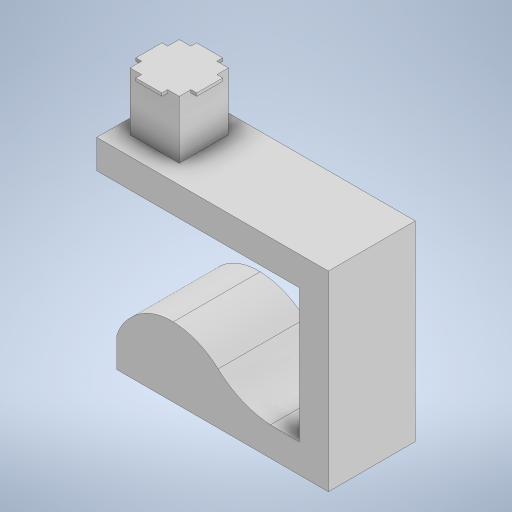
# Autodesk Inventor part: GroundClipV1
Saved by Autodesk Inventor 2024.2 (Build 282272000, 272)
## iProperties
Created: 2024-01-05
Part Number: GroundClipV1
Material: Generic
Document SubType Name: Modeling
Designer: chris
Density: 1 g/cm^3
Appearance: Default
Author: chris
Autodesk Inventor part; units mm, degrees
ref_plane "YZ Plane" through (0, 0, 0) normal (1, 0, 0) x (0, 1, 0)
ref_plane "XZ Plane" through (0, 0, 0) normal (0, 1, 0) x (-1, 0, 0)
ref_plane "XY Plane" through (0, 0, 0) normal (0, 0, 1) x (1, 0, 0)
sketch "Sketch1" plane through (0, 0, 0) normal (0, 1, 0) x (-1, 0, 0)
  line L0 (-20, -7.5) -> (20, -7.5)
  line L1 (20, -7.5) -> (20, 7.5)
  line L2 (20, 7.5) -> (-20, 7.5)
  line L3 (-20, 7.5) -> (-20, -7.5)
  line L4 (-20, -7.5) -> (20, 7.5) construction
  line L5 (20, -7.5) -> (-20, 7.5) construction
  point P0 (0, 0)
  dimension "d0" = 15
  dimension "d1" = 40
  constraints: 12 end point, 2 midpoint, 2 parallel, 1 horizontal, 1 perpendicular
  measures "d0" distance of L0.end L1.end
  measures "d1" distance between parallel lines of L3 L1
extrude "Extrusion1" add sketch "Sketch1" along normal blind 5
sketch "Sketch2" plane through (20, 0, 7.5) normal (1, 0, 0) x (0, 0, -1)
  line L0 (15, 0) -> (0, 0) projected
  line L1 (0, -28) -> (0, 0)
  line L2 (15, 0) -> (15, -28)
  line L3 (15, -28) -> (0, -28)
  line L4 (0, 0) -> (15, 0) projected
  line L5 (15, 0) -> (0, 0)
  point P0 (7.5, 0)
  dimension "d13" = 28
  constraints: 8 end point, 1 collinear, 1 perpendicular, 1 vertical
  measures "d13" distance of L0.start L2.end
extrude "Extrusion2" add sketch "Sketch2" against normal blind 5
sketch "Sketch3" plane through (-20, 5, 7.5) normal (0, 0, 1) x (1, 0, 0)
  line L0 (35, -5) -> (35, -33) projected
  line L1 (35, -33) -> (30, -33)
  line L2 (35, -28) -> (30, -28)
  line L3 (35, -25) -> (-4.3646, -25) construction
  line L4 (0, -5) -> (35, -5) construction
  line L5 (30, -33) -> (3.4423, -33)
  line L6 (35, -21) -> (-4.3646, -21) construction
  line L7 (3.4423, -33) -> (21.0714, -33)
  arc A0 (20.9558, -24.1562) -> (30, -28) centre (30.8945, -13.3333) ccw
  arc A1 (20.9558, -24.1562) -> (13.2077, -21) centre (12.838, -32.9961) ccw
  arc A2 (13.2077, -21) -> (5.7637, -24.1543) centre (12.91, -30.6583) ccw
  arc A3 (5.7637, -24.1543) -> (3.4423, -28) centre (11.7993, -30.4211) ccw
  line L8 (3.4423, -33) -> (3.4423, -28)
  point P0 (20, -5)
  point P1 (35, -5)
  dimension "d7" = 5
  dimension "d8" = 5
  dimension "d9" = 20
  dimension "d10" = 4
  constraints: 14 end point, 8 point on circle, 6 horizontal, 4 centre point, 4 point on line, 2 tangent, 1 vertical
  measures "d7" distance of L0.end L1.end
  measures "d8" distance between parallel lines of L2 L1
  measures "d9" distance between parallel lines of L3 L4
  measures "d10" distance between parallel lines of L6 L3
extrude "Extrusion3" add sketch "Sketch3" against normal up to surface (15 mm away)
sketch "Sketch4" plane through (0, 5, 0) normal (0, 1, 0) x (1, 0, 0)
  line L0 (-17.5, 4.25) -> (-9, 4.25)
  line L1 (-9, 4.25) -> (-9, -4.25)
  line L2 (-9, -4.25) -> (-17.5, -4.25)
  line L3 (-17.5, -4.25) -> (-17.5, 4.25)
  line L4 (-20, 7.5) -> (-20, -7.5) projected
  point P0 (0, 0)
  dimension "d14" = 8.5
  dimension "d15" = 2.5
  dimension "d16" = 4.25
  dimension "d17" = 4.25
  constraints: 8 end point, 2 parallel, 1 horizontal, 1 perpendicular
  measures "d14" distance of L0.start L0.end
  measures "d15" distance between parallel lines of L4 L3
  measures "d16" distance from line of point (0, 0) L0
  measures "d17" distance from line of point (0, 0) L2
extrude "Extrusion4" add sketch "Sketch4" along normal blind 10
sketch "Sketch5" plane through (0, 15, 0) normal (0, 1, 0) x (1, 0, 0)
  line L0 (-17.5, 4.25) -> (-9, 4.25) projected
  line L1 (-15.5, 4.25) -> (-11, 4.25)
  line L2 (-11, 4.25) -> (-11, 5.25)
  line L3 (-11, 5.25) -> (-15.5, 5.25)
  line L4 (-15.5, 5.25) -> (-15.5, 4.25)
  line L5 (-9, -4.25) -> (-9, 4.25) projected
  line L6 (-17.5, 4.25) -> (-17.5, -4.25) projected
  point P0 (0, 0)
  dimension "d20" = 2
  dimension "d21" = 2
  dimension "d22" = 1
  constraints: 8 end point, 2 parallel, 1 horizontal, 1 perpendicular, 1 point on line
  measures "d20" distance between parallel lines of L2 L5
  measures "d21" distance between parallel lines of L6 L4
  measures "d22" distance between parallel lines of L0 L3
extrude "Extrusion5" add sketch "Sketch5" against normal blind 0.5
sketch "Sketch6" plane through (0, 15, 0) normal (0, 1, 0) x (1, 0, 0)
  line L0 (-17.5, 4.25) -> (-9, 4.25) construction
  line L1 (-9, -4.25) -> (-9, 4.25) construction
  line L2 (-17.5, 4.25) -> (-9, -4.25) construction
  line L3 (-9, 4.25) -> (-17.5, -4.25) construction
  point P0 (0, 0)
  point P1 (-13.25, 0)
  constraints: 4 end point, 1 midpoint
pattern_circular "Circular Pattern1" count 4 over 360 about axis through (-13.25, 15, 0) along (0, 1, 0) of "Extrusion5"
equation "\"d16\" = 0.5 * d14"
equation "\"d17\" = 0.5 * d14"
body "Solid1"
